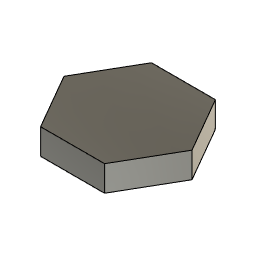
Hexagonal_Prism (Autodesk Fusion 360 design; units mm, degrees)
Autodesk Fusion 360 part; units mm, degrees
sketch "Hexagon" plane through (0, 0, 0) normal (0, 0, 1) x (1, 0, 0)
  line L0 (0, 0) -> (50, 0)
  line L1 (50, 0) -> (75, 43.3013)
  line L2 (75, 43.3013) -> (50, 86.6025)
  line L3 (50, 86.6025) -> (0, 86.6025)
  line L4 (0, 86.6025) -> (-25, 43.3013)
  line L5 (-25, 43.3013) -> (0, 0)
  line L6 (0, 0) -> (50, 0) construction
  point P0 (25, 43.3013)
  dimension "d1" = 50
  dimension "d2" = 0
  dimension "d3" = 86.6025
  dimension "d4" = 100
  constraint coincident L0.start L5.end
  constraint horizontal L6
  measures "d1" distance of L0.start L0.end
  measures "d2" angle of L0 L6
  measures "d3" distance of L0 L3
  measures "d4" distance of L1.end L4.end
extrude "Extrude1" add sketch "Hexagon" along normal blind 20
named bodies: "Hexagon"
